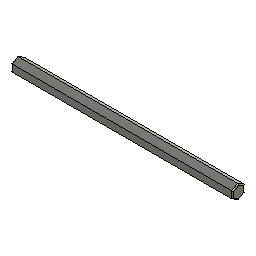
main_driver (Autodesk Fusion 360 design; units mm, degrees)
part number: 2026-05-19-16-10-02-554
Autodesk Fusion 360 part; units mm, degrees
sketch "main_driver" plane through (0, 0, 0) normal (1, 0, 0) x (0, 1, 0)
  line L0 (150, 45.3) -> (154.0703, 47.65)
  line L1 (154.0703, 47.65) -> (154.0703, 52.35)
  line L2 (154.0703, 52.35) -> (150, 54.7)
  line L3 (150, 54.7) -> (145.9297, 52.35)
  line L4 (145.9297, 52.35) -> (145.9297, 47.65)
  line L5 (145.9297, 47.65) -> (150, 45.3)
  point P0 (150, 50)
  dimension "d1" = 4.7
  measures "d1" distance of L0.start P0
extrude "Extrude1" add sketch "main_driver" against normal blind 150
fillet "Fillet1" radius 0.75 12 edges at (-150, 147.9648, 53.525) (-150, 152.0352, 53.525) (-150, 154.0703, 50) (-150, 152.0352, 46.475) (-150, 147.9648, 46.475) (-150, 145.9297, 50) (0, 152.0352, 53.525) (0, 147.9648, 53.525) (0, 145.9297, 50) (0, 147.9648, 46.475) (0, 152.0352, 46.475) (0, 154.0703, 50)
named bodies: "main_driver"
